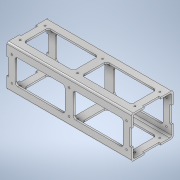
# Autodesk Inventor part: MainPart1
Saved by Autodesk Inventor 2022 (Build 260153000, 153)
## iProperties
Created: 2022-04-04
Part Number: MainPart1
Material: Aluminum 6061, Welded
Document SubType Name: Modeling
Designer: ForseFire
Density: 2.7 g/cm^3
Appearance: Aluminum - Polished
Author: ForseFire
Autodesk Inventor part; units mm, degrees
ref_plane "YZ Plane" through (0, 0, 0) normal (1, 0, 0) x (0, 1, 0)
ref_plane "XZ Plane" through (0, 0, 0) normal (0, 1, 0) x (-1, 0, 0)
ref_plane "XY Plane" through (0, 0, 0) normal (0, 0, 1) x (1, 0, 0)
sketch "Sketch1" plane through (0, 0, 0) normal (1, 0, 0) x (0, 1, 0)
  line L0 (-25, -25) -> (25, -25)
  line L1 (25, -25) -> (25, 25)
  line L2 (25, 25) -> (-25, 25)
  line L3 (-25, 25) -> (-25, -25)
  line L4 (-25, -25) -> (25, 25) construction
  line L5 (25, -25) -> (-25, 25) construction
  line L6 (-23, 23) -> (23, 23)
  line L7 (23, 23) -> (23, -23)
  line L8 (23, -23) -> (-23, -23)
  line L9 (-23, -23) -> (-23, 23)
  line L10 (-23, 23) -> (23, -23) construction
  line L11 (23, 23) -> (-23, -23) construction
  point P0 (0, 0)
  dimension "d0" = 50
  dimension "d1" = 50
  dimension "d2" = 46
  dimension "d3" = 46
  constraints: 24 end point, 4 midpoint, 4 parallel, 2 horizontal, 2 perpendicular, 1 point on line
  measures "d0" distance of L1.end L2.end
  measures "d1" distance of L0.end L1.end
  measures "d2" distance of L6.end L7.end
  measures "d3" distance of L6.start L6.end
extrude "Extrusion1" add sketch "Sketch1" along normal blind 150
sketch "Sketch2" plane through (0, 0, 0) normal (-1, 0, 0) x (0, 0, 1)
  line L0 (-23, 23) -> (-23, -23) projected
  line L1 (-23, 0) -> (-25, 0)
  line L2 (-25, -25) -> (-25, 25) projected
  line L3 (23, 23) -> (-23, 23) projected
  line L4 (0, 23) -> (0, 25)
  line L5 (-25, 25) -> (25, 25) projected
  line L6 (23, -23) -> (23, 23) projected
  line L7 (23, 0) -> (25, 0)
  line L8 (25, 25) -> (25, -25) projected
  line L9 (-23, -23) -> (23, -23) projected
  line L10 (0, -23) -> (0, -25)
  line L11 (25, -25) -> (-25, -25) projected
  line L12 (-23, -10) -> (-25, -10)
  line L13 (-25, -10) -> (-25, 10)
  line L14 (-25, 10) -> (-23, 10)
  line L15 (-23, 10) -> (-23, -10)
  line L16 (-23, -10) -> (-25, 10) construction
  line L17 (-25, -10) -> (-23, 10) construction
  line L18 (10, 23) -> (-10, 23)
  line L19 (-10, 23) -> (-10, 25)
  line L20 (-10, 25) -> (10, 25)
  line L21 (10, 25) -> (10, 23)
  line L22 (10, 23) -> (-10, 25) construction
  line L23 (-10, 23) -> (10, 25) construction
  line L24 (23, -10) -> (25, -10)
  line L25 (25, -10) -> (25, 10)
  line L26 (25, 10) -> (23, 10)
  line L27 (23, 10) -> (23, -10)
  line L28 (23, -10) -> (25, 10) construction
  line L29 (25, -10) -> (23, 10) construction
  line L30 (10, -23) -> (-10, -23)
  line L31 (-10, -23) -> (-10, -25)
  line L32 (-10, -25) -> (10, -25)
  line L33 (10, -25) -> (10, -23)
  line L34 (10, -23) -> (-10, -25) construction
  line L35 (-10, -23) -> (10, -25) construction
  point P0 (0, 0)
  point P1 (-24, 0)
  point P2 (0, 24)
  point P3 (24, 0)
  point P4 (0, -24)
  point P5 (10, 25)
  point P6 (-10, 23)
  dimension "d6" = 20
  dimension "d7" = 20
  dimension "d8" = 20
  dimension "d9" = 20
  constraints: 56 end point, 20 midpoint, 8 parallel, 4 horizontal, 4 perpendicular, 4 point on line
  measures "d6" distance between parallel lines of L12 L14
  measures "d7" distance between parallel lines of L21 L19
  measures "d8" distance between parallel lines of L24 L26
  measures "d9" distance between parallel lines of L33 L31
extrude "Extrusion2" cut sketch "Sketch2" against normal blind 2 contours L0 L1 L2 L14 | L19 L5 L4 L3 | L0 L12 L2 L1 | L4 L5 L21 L3 | L9 L10 L11 L31 | L26 L8 L7 L6 | L9 L33 L11 L10 | L7 L8 L24 L6
sketch "Sketch3" plane through (150, 0, 0) normal (1, 0, 0) x (0, 0, -1)
  line L0 (25, -10) -> (25, 10) projected
  line L1 (25, 0) -> (23, 0)
  line L2 (23, 23) -> (23, -23) projected
  line L3 (-10, 23) -> (10, 23) projected
  line L4 (0, 23) -> (0, 25)
  line L5 (10, 25) -> (-10, 25) projected
  line L6 (-25, -25) -> (25, -25) projected
  line L7 (0, -25) -> (0, -23)
  line L8 (23, -23) -> (-23, -23) projected
  line L9 (-23, -23) -> (-23, 23) projected
  line L10 (-23, 0) -> (-25, 0)
  line L11 (-25, 10) -> (-25, -10) projected
  line L12 (-25, -10) -> (-23, -10)
  line L13 (-23, -10) -> (-23, 10)
  line L14 (-23, 10) -> (-25, 10)
  line L15 (-25, 10) -> (-25, -10)
  line L16 (-25, -10) -> (-23, 10) construction
  line L17 (-23, -10) -> (-25, 10) construction
  line L18 (-10, -23) -> (10, -23)
  line L19 (10, -23) -> (10, -25)
  line L20 (10, -25) -> (-10, -25)
  line L21 (-10, -25) -> (-10, -23)
  line L22 (-10, -23) -> (10, -25) construction
  line L23 (10, -23) -> (-10, -25) construction
  line L24 (23, 10) -> (25, 10)
  line L25 (25, 10) -> (25, -10)
  line L26 (25, -10) -> (23, -10)
  line L27 (23, -10) -> (23, 10)
  line L28 (23, 10) -> (25, -10) construction
  line L29 (25, 10) -> (23, -10) construction
  line L30 (-10, 23) -> (10, 23)
  line L31 (10, 23) -> (10, 25)
  line L32 (10, 25) -> (-10, 25)
  line L33 (-10, 25) -> (-10, 23)
  line L34 (-10, 23) -> (10, 25) construction
  line L35 (10, 23) -> (-10, 25) construction
  point P0 (0, 0)
  point P1 (-24, 0)
  point P2 (0, -24)
  point P3 (24, 0)
  point P4 (0, 24)
  point P5 (10, -23)
  dimension "d12" = 20
  dimension "d13" = 20
  dimension "d14" = 20
  dimension "d15" = 20
  constraints: 56 end point, 20 midpoint, 8 parallel, 4 horizontal, 4 perpendicular, 4 point on line
  measures "d12" distance between parallel lines of L12 L14
  measures "d13" distance between parallel lines of L21 L19
  measures "d14" distance between parallel lines of L26 L24
  measures "d15" distance between parallel lines of L33 L31
extrude "Extrusion3" cut sketch "Sketch3" against normal blind 2
sketch "Sketch4" plane through (0, 25, -25) normal (0, 1, 0) x (1, 0, 0)
  line L0 (0, -50) -> (150, -50) projected
  line L1 (0, 0) -> (150, 0) projected
  line L2 (40, 0) -> (110, 0)
  line L3 (110, 0) -> (110, -50)
  line L4 (110, -50) -> (40, -50)
  line L5 (40, -50) -> (40, 0)
  line L6 (40, 0) -> (110, -50) construction
  line L7 (110, 0) -> (40, -50) construction
  line L8 (10, -10) -> (70, -10)
  line L9 (70, -10) -> (70, -40)
  line L10 (70, -40) -> (10, -40)
  line L11 (10, -40) -> (10, -10)
  line L12 (10, -10) -> (70, -40) construction
  line L13 (70, -10) -> (10, -40) construction
  line L14 (80, -10) -> (140, -10)
  line L15 (140, -10) -> (140, -40)
  line L16 (140, -40) -> (80, -40)
  line L17 (80, -40) -> (80, -10)
  line L18 (80, -10) -> (140, -40) construction
  line L19 (140, -10) -> (80, -40) construction
  line L20 (0, 0) -> (0, -15) projected
  line L21 (150, -35) -> (150, -50) projected
  point P0 (0, -25)
  point P1 (75, -25)
  point P2 (40, -25)
  point P3 (110, -25)
  dimension "d19" = 60
  dimension "d20" = 30
  dimension "d21" = 60
  dimension "d22" = 30
  dimension "d77" = 40
  dimension "d78" = 40
  constraints: 36 end point, 8 midpoint, 6 parallel, 3 horizontal, 3 perpendicular, 1 point on line
  measures "d19" distance of L9.end L10.end
  measures "d20" distance of L8.end L9.end
  measures "d21" distance of L15.end L16.end
  measures "d22" distance of L14.end L15.end
  measures "d77" distance between parallel lines of L20 L5
  measures "d78" distance between parallel lines of L21 L3
extrude "Extrusion4" cut sketch "Sketch4" against normal through all contours L10 L11 L8 L5 | L5 L8 L9 L10 | L16 L17 L14 L3 | L3 L14 L15 L16
sketch "Sketch7" plane through (0, 25, 25) normal (0, 0, 1) x (1, 0, 0)
  line L0 (0, -50) -> (150, -50) projected
  line L1 (0, 0) -> (150, 0) projected
  line L2 (40, 0) -> (110, 0)
  line L3 (110, 0) -> (110, -50)
  line L4 (110, -50) -> (40, -50)
  line L5 (40, -50) -> (40, 0)
  line L6 (40, 0) -> (110, -50) construction
  line L7 (110, 0) -> (40, -50) construction
  line L8 (80, -10) -> (140, -10)
  line L9 (140, -10) -> (140, -40)
  line L10 (140, -40) -> (80, -40)
  line L11 (80, -40) -> (80, -10)
  line L12 (80, -10) -> (140, -40) construction
  line L13 (140, -10) -> (80, -40) construction
  line L14 (10, -10) -> (70, -10)
  line L15 (70, -10) -> (70, -40)
  line L16 (70, -40) -> (10, -40)
  line L17 (10, -40) -> (10, -10)
  line L18 (10, -10) -> (70, -40) construction
  line L19 (70, -10) -> (10, -40) construction
  line L20 (0, 0) -> (0, -15) projected
  line L21 (150, 0) -> (150, -15) projected
  point P0 (0, -25)
  point P1 (75, -25)
  point P2 (110, -25)
  point P3 (40, -25)
  dimension "d26" = 50
  dimension "d27" = 60
  dimension "d28" = 30
  dimension "d29" = 60
  dimension "d30" = 30
  dimension "d117" = 40
  dimension "d118" = 40
  constraints: 36 end point, 8 midpoint, 6 parallel, 3 horizontal, 3 perpendicular
  measures "d26" distance of L2.end L3.end
  measures "d27" distance of L9.end L10.end
  measures "d28" distance of L8.end L9.end
  measures "d29" distance of L15.end L16.end
  measures "d30" distance of L16.end L14.start
  measures "d117" distance between parallel lines of L5 L20
  measures "d118" distance between parallel lines of L3 L21
extrude "Extrusion5" cut sketch "Sketch7" against normal through all contours L16 L17 L14 L5 | L5 L14 L15 L16 | L10 L11 L8 L3 | L3 L8 L9 L10
sketch "Sketch19" plane through (0, 25, -25) normal (0, 1, 0) x (1, 0, 0)
  line L0 (0, -15) -> (2, -15) projected
  line L1 (1.5, 0) -> (3.5, 0) projected
  line L2 (2, -15) -> (2, -35) projected
  line L3 (2, -50) -> (2, -48) projected
  line L4 (150, -35) -> (148, -35) projected
  line L5 (0, -50) -> (150, -50) projected
  line L6 (148, -15) -> (150, -15) projected
  line L7 (0, 0) -> (150, 0) projected
  line L8 (1.5, -50) -> (1.5, -48) projected
  line L9 (2.5, -35) -> (1.5, -35)
  line L10 (1.5, -50) -> (2.5, -50)
  line L11 (2.5, 0) -> (1.5, 0)
  line L12 (1.5, -15) -> (2.5, -15)
  line L13 (148.5, 0) -> (147.5, 0)
  line L14 (147.5, -15) -> (148.5, -15)
  line L15 (148.5, -35) -> (147.5, -35)
  line L16 (147.5, -50) -> (148.5, -50)
  circle A0 centre (6, -10) radius 1
  line L17 (0, 0) -> (0, -15) projected
  circle A1 centre (6, -40) radius 1
  line L18 (0, -35) -> (0, -50) projected
  circle A2 centre (144, -40) radius 1
  line L19 (150, -35) -> (150, -50) projected
  circle A3 centre (144, -10) radius 1
  line L20 (150, 0) -> (150, -15) projected
  circle A4 centre (75, -40) radius 1
  line L21 (70, -10) -> (70, -40) projected
  circle A5 centre (75, -10) radius 1
  point P0 (0, -25)
  dimension "d79" = 2
  dimension "d80" = 6
  dimension "d81" = 10
  dimension "d82" = 2
  dimension "d83" = 6
  dimension "d84" = 10
  dimension "d85" = 2
  dimension "d86" = 6
  dimension "d87" = 10
  dimension "d88" = 2
  dimension "d89" = 6
  dimension "d90" = 10
  dimension "d105" = 2
  dimension "d106" = 10
  dimension "d107" = 5
  dimension "d108" = 2
  dimension "d109" = 10
  dimension "d110" = 5
  constraints: 16 end point, 6 centre point, 5 point on line, 4 horizontal, 4 parallel
  measures "d79" diameter of A0
  measures "d80" distance from line of A0.centre L17
  measures "d81" distance from line of A0.centre L7
  measures "d82" diameter of A1
  measures "d83" distance from line of A1.centre L18
  measures "d84" distance from line of A1.centre L5
  measures "d85" diameter of A2
  measures "d86" distance from line of A2.centre L19
  measures "d87" distance from line of A2.centre L5
  measures "d88" diameter of A3
  measures "d89" distance from line of A3.centre L20
  measures "d90" distance from line of A3.centre L7
  measures "d105" diameter of A4
  measures "d106" distance from line of A4.centre L5
  measures "d107" distance from line of A4.centre L21
  measures "d108" diameter of A5
  measures "d109" distance from line of A5.centre L7
  measures "d110" distance from line of A5.centre L21
extrude "Extrusion14" cut sketch "Sketch19" against normal through all
sketch "Sketch21" plane through (0, 25, 25) normal (0, 0, 1) x (1, 0, 0)
  circle A0 centre (6, -40) radius 1
  line L0 (0, -48) -> (0, -35) projected
  line L1 (0, -50) -> (150, -50) projected
  circle A1 centre (6, -10) radius 1
  line L2 (0, 0) -> (0, -15) projected
  line L3 (0, 0) -> (150, 0) projected
  circle A2 centre (144, -10) radius 1
  line L4 (150, 0) -> (150, -15) projected
  circle A3 centre (144, -40) radius 1
  line L5 (150, -35) -> (150, -50) projected
  circle A4 centre (75, -10) radius 1
  line L6 (70, -10) -> (70, -40) projected
  circle A5 centre (75, -40) radius 1
  point P0 (0, -25)
  dimension "d91" = 2
  dimension "d92" = 6
  dimension "d93" = 10
  dimension "d94" = 2
  dimension "d95" = 6
  dimension "d96" = 10
  dimension "d97" = 2
  dimension "d98" = 10
  dimension "d99" = 6
  dimension "d100" = 2
  dimension "d101" = 6
  dimension "d102" = 10
  dimension "d111" = 2
  dimension "d112" = 5
  dimension "d113" = 10
  dimension "d114" = 2
  dimension "d115" = 10
  dimension "d116" = 5
  constraints: 6 centre point
  measures "d91" diameter of A0
  measures "d92" distance from line of L0 A0.centre
  measures "d93" distance from line of A0.centre L1
  measures "d94" diameter of A1
  measures "d95" distance from line of A1.centre L2
  measures "d96" distance from line of A1.centre L3
  measures "d97" diameter of A2
  measures "d98" distance from line of A2.centre L3
  measures "d99" distance from line of A2.centre L4
  measures "d100" diameter of A3
  measures "d101" distance from line of A3.centre L5
  measures "d102" distance from line of A3.centre L1
  measures "d111" diameter of A4
  measures "d112" distance from line of A4.centre L6
  measures "d113" distance from line of A4.centre L3
  measures "d114" diameter of A5
  measures "d115" distance from line of A5.centre L1
  measures "d116" distance from line of A5.centre L6
extrude "Extrusion15" cut sketch "Sketch21" against normal through all
fillet "Fillet1" radius 3 32 edges at (10, -24, 15) (10, -24, -15) (70, -24, -15) (70, -24, 15) (80, -24, 15) (80, -24, -15) (140, -24, -15) (140, -24, 15) (10, -15, 24) (10, 15, 24) (10, 24, -15) (70, 15, 24) (70, 24, -15) (70, 15, -24) (70, -15, 24) (70, -15, -24) (140, -15, -24) (140, -15, 24) (140, 15, 24) (140, 15, -24) (140, 24, -15) (10, -15, -24) (70, 24, 15) (10, 24, 15) (80, 24, 15) (80, 24, -15) (80, -15, -24) (140, 24, 15) (80, -15, 24) (80, 15, 24) (80, 15, -24) (10, 15, -24)
fillet "Fillet2" radius 2 8 edges at (75, 23, 23) (75, 25, 25) (75, 23, -23) (75, 25, -25) (75, -25, 25) (75, -23, 23) (75, -23, -23) (75, -25, -25)
body "Solid1"
